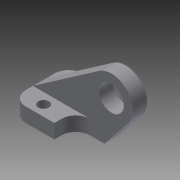
# Autodesk Inventor part: HW 6 Part 4
Saved by Autodesk Inventor 2015 (Build 190159000, 159)
## iProperties
Created: 2016-02-13
Part Number: HW 6 Part 4
Material: Generic
Document SubType Name: Modeling
Designer: Melissa
Density: 1 g/cm^3
Appearance: Default
Author: Melissa
Autodesk Inventor part; units mm, degrees
ref_plane "YZ Plane" through (0, 0, 0) normal (1, 0, 0) x (0, 1, 0)
ref_plane "XZ Plane" through (0, 0, 0) normal (0, 1, 0) x (-1, 0, 0)
ref_plane "XY Plane" through (0, 0, 0) normal (0, 0, 1) x (1, 0, 0)
sketch "Sketch1" plane through (0, 0, 0) normal (0, 0, 1) x (1, 0, 0)
  arc A0 (29.6299, -23.9516) -> (-21.7746, 31.2646) centre (0, 0) ccw
  circle A1 centre (0, 0) radius 22.225
  line L0 (-21.7746, 31.2646) -> (-139.6057, -50.8)
  line L1 (-139.6057, -50.8) -> (-139.6057, -76.2)
  line L2 (-139.6057, -76.2) -> (-12.6057, -76.2)
  line L3 (-12.6057, -76.2) -> (29.6299, -23.9516)
  dimension "d0" = 76.2
  dimension "d1" = 44.45
  dimension "d2" = 25.4
  dimension "d3" = 76.2
  dimension "d4" = 127
  constraints: 8 end point, 2 centre point, 2 coincident, 2 point on circle, 2 tangent, 1 perpendicular, 1 vertical
  measures "d0" diameter of A0
  measures "d1" diameter of A1
  measures "d2" distance of L0.end L1.end
  measures "d3" vertical distance of L2.end point (0, 0)
  measures "d4" distance of L1.end L2.end
extrude "Extrusion1" add sketch "Sketch1" along normal blind 25.4
sketch "Sketch2" plane through (-139.6057, -76.2, 0) normal (0, -1, 0) x (1, 0, 0)
  line L0 (0, 0) -> (0, 25.4) projected
  line L1 (0, 12.7) -> (0, 38.1)
  line L2 (25.4, 63.5) -> (76.2, 63.5)
  line L3 (76.2, -25.4) -> (76.2, -38.1)
  line L4 (76.2, -38.1) -> (25.4, -38.1)
  line L5 (0, -12.7) -> (0, 12.7)
  arc A0 (25.4, 63.5) -> (0, 38.1) centre (25.4, 38.1) ccw
  arc A1 (0, -12.7) -> (25.4, -38.1) centre (25.4, -12.7) ccw
  circle A2 centre (38.1, -19.05) radius 9.525
  circle A3 centre (38.1, 44.45) radius 9.525
  line L6 (101.6, 0) -> (100.5996, 0)
  line L7 (0, 0) -> (117.8311, 0) projected
  arc A4 (101.6, 0) -> (76.2, -25.4) centre (101.6, -25.4) ccw
  line L8 (76.2, 63.5) -> (76.2, 50.8)
  line L9 (101.6, 25.4) -> (97.5099, 25.4)
  line L10 (117.8311, 25.4) -> (0, 25.4) projected
  arc A5 (76.2, 50.8) -> (101.6, 25.4) centre (101.6, 50.8) ccw
  line L11 (101.6, 25.4) -> (101.6, 0)
  point P0 (139.6057, 0)
  point P1 (0, 63.5)
  point P2 (0, -38.1)
  dimension "d7" = 50.8
  dimension "d8" = 76.2
  dimension "d9" = 101.6
  dimension "d10" = 25.4
  dimension "d11" = 19.05
  dimension "d12" = 19.05
  dimension "d13" = 38.1
  dimension "d16" = 25.4
  dimension "d17" = 25.4
  constraints: 18 end point, 8 point on circle, 8 point on line, 8 tangent, 6 centre point, 3 perpendicular, 3 vertical, 1 collinear, 1 equal radius, 1 midpoint
  measures "d7" distance of L1.start point (0, 63.5)
  measures "d8" distance of point (0, 63.5) L2.end
  measures "d9" distance of L2.end L3.end
  measures "d10" radius of A0
  measures "d11" diameter of A2
  measures "d12" distance from line of L4 A2.centre
  measures "d13" distance from line of L5 A2.centre
  measures "d16" radius of A4
  measures "d17" radius of A5
extrude "Extrusion2" add sketch "Sketch2" against normal blind 25.4
body "Solid1"
